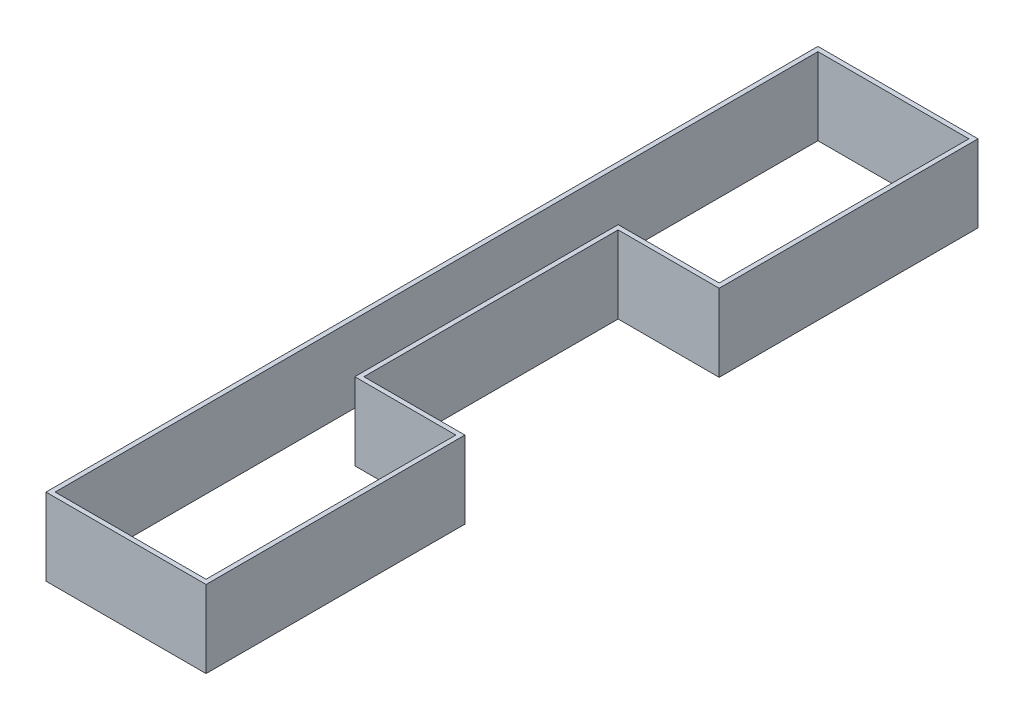
# Autodesk Inventor part: farbian isch an pfoschten
Saved by Autodesk Inventor 2021 (Build 250183000, 183)
## iProperties
Created: 2021-11-30
Part Number: farbian isch an pfoschten
Material: Generisch
Document SubType Name: Modeling
Designer: Fabian
Density: 1 g/cm^3
Appearance: Vorgabe
Author: Fabian
Autodesk Inventor part; units mm, degrees
ref_plane "XZ Plane" through (0, 0, 0) normal (0, 1, 0) x (-1, 0, 0)
sketch "Skizze1" plane through (0, 0, 0) normal (0, 1, 0) x (-1, 0, 0)
  line L0 (0, 0) -> (0, 112)
  line L1 (0, 112) -> (-89, 112)
  line L2 (0, 0) -> (0, -112)
  line L3 (0, -112) -> (-89, -112)
  line L4 (-89, -112) -> (-89, -340)
  line L5 (-89, 340) -> (52, 340)
  line L6 (52, 340) -> (52, -340)
  line L7 (52, -340) -> (-89, -340)
  line L8 (-89, 116) -> (4, 116)
  line L9 (4, 116) -> (4, -116)
  line L10 (4, -116) -> (-89, -116)
  line L11 (-85, -116) -> (-85, -336)
  line L12 (-89, -336) -> (52, -336)
  line L13 (-85, 116) -> (-85, 336)
  line L14 (48, 336) -> (48, -336)
  line L15 (52, 336) -> (-89, 336)
  line L16 (-89, 340) -> (-89, 336)
  line L17 (-89, 116) -> (-89, 336)
  line L18 (-89, 116) -> (-89, 112)
  line L19 (0, 112) -> (4, 116)
  line L20 (0, -112) -> (4, -116)
  dimension "d1" = 89
  dimension "d4" = 89
  dimension "d5" = 228
  dimension "d6" = 141
  dimension "d7" = 4
  dimension "d8" = 4
  dimension "d9" = 4
  dimension "d21" = 224
  dimension "d22" = 4
  dimension "d23" = 4
  dimension "d24" = 220
  dimension "d28" = 4
  constraints: 42 end point, 8 perpendicular, 7 point on line, 4 vertical, 3 horizontal, 2 collinear, 1 parallel
  measures "d1" distance of L0.end L1.end
  measures "d4" distance of L2.end L3.end
  measures "d5" distance of L3.end L4.end
  measures "d6" distance of L5.start L5.end
  measures "d7" distance between parallel lines of L1 L8
  measures "d8" distance between parallel lines of L0 L9
  measures "d9" distance between parallel lines of L3 L10
  measures "d21" distance of L2.end L0.end
  measures "d22" distance between parallel lines of L4 L11
  measures "d23" distance between parallel lines of L7 L12
  measures "d24" distance of L11.start L11.end
  measures "d28" distance between parallel lines of L6 L14
ref_plane "Arbeitsebene1" through (0, 0, 112) normal (0, 0, 1) x (1, 0, 0)
ref_plane "Arbeitsebene2" through (0, 0, -112) normal (0, 0, 1) x (1, 0, 0)
sketch "Skizze2" plane through (0, 0, 112) normal (0, 0, 1) x (1, 0, 0)
  line L0 (0, 0) -> (0, -68)
  line L1 (0, -68) -> (89, -68)
  line L2 (89, -68) -> (89, 0)
  line L3 (89, 0) -> (0, 0)
  dimension "d12" = 68
  dimension "d13" = 89
  constraints: 8 end point, 3 perpendicular, 1 vertical
  measures "d12" distance of L0.start L0.end
  measures "d13" distance of L0.end L1.end
sketch "Skizze3" plane through (0, 0, -112) normal (0, 0, 1) x (1, 0, 0)
  line L0 (0, 0) -> (89, 0)
  line L1 (89, 0) -> (89, -68)
  line L2 (89, -68) -> (0, -68)
  line L3 (0, -68) -> (0, 0)
  dimension "d14" = 89
  dimension "d15" = 68
  constraints: 8 end point, 2 perpendicular, 1 horizontal
  measures "d14" distance of L0.start L0.end
  measures "d15" distance of L0.end L1.end
derived "Mastersketch.ipt"
sketch "Skizze4" plane through (0, 0, 0) normal (1, 0, 0) x (0, 1, 0)
  point P0 (0, 0)
extrude "Extrusion1" add sketch "Skizze1" against normal blind 68 contours L0 L19 L9 L20 L2 | L1 L18 L8 L19 | L20 L10 L4 L3 | L17 L15 L13 L8 | L10 L11 L12 L4 | L16 L5 L6 L15 | L12 L6 L7 L4 | L15 L6 L12 L14
equation "\"d1\" = goal_depth"
equation "\"d4\" = goal_depth"
equation "\"d5\" = goalPlayArea_distance"
equation "\"d6\" = goalPanelSideOuter_width"
equation "\"d7\" = goalPanel_thickness"
equation "\"d8\" = goalPanel_thickness"
equation "\"d9\" = goalPanel_thickness"
equation "\"d21\" = goal_width"
equation "\"d22\" = goalPanel_thickness"
equation "\"d23\" = goalPanel_thickness"
equation "\"d24\" = goalPanelFrontInner_innerWidth"
equation "\"d28\" = goalPanel_thickness"
equation "\"d12\" = goalCollector_depth"
equation "\"d14\" = goal_depth"
equation "\"d15\" = goalCollector_depth"
equation "\"goal_depth\" = 89"
equation "\"goalPlayArea_distance\" = 228"
equation "\"goalPanelSideOuter_width\" = 141"
equation "\"goalPanel_thickness\" = 4"
equation "\"goal_width\" = 224"
equation "\"goalPanelFrontInner_innerWidth\" = 220"
equation "\"goalCollector_depth\" = 68"
